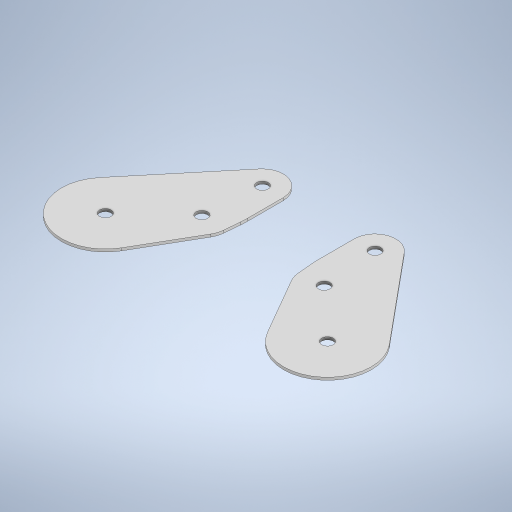
# Autodesk Inventor part: IntakeHolderTopPlate
Saved by Autodesk Inventor 2023 (Build 270158000, 158)
## iProperties
Created: 2022-09-11
Part Number: IntakeHolderTopPlate
Material: Generic
Document SubType Name: Modeling
Designer: deli
Density: 1 g/cm^3
Appearance: Default
Author: deli
Autodesk Inventor part; units mm, degrees
ref_plane "YZ Plane" through (0, 0, 0) normal (1, 0, 0) x (0, 1, 0)
ref_plane "XZ Plane" through (0, 0, 0) normal (0, 1, 0) x (-1, 0, 0)
ref_plane "XY Plane" through (0, 0, 0) normal (0, 0, 1) x (1, 0, 0)
sketch "Sketch1" plane through (0, 0, 0) normal (0, 1, 0) x (-1, 0, 0)
  circle A0 centre (21.4316, 162.4913) radius 7
  circle A1 centre (21.4316, 162.4913) radius 24 construction
  circle A2 centre (15.5486, 229.7344) radius 24 construction
  circle A3 centre (15.5486, 229.7344) radius 7
  circle A4 centre (157.4316, 162.4913) radius 7
  circle A5 centre (163.3146, 229.7344) radius 7
  circle A6 centre (163.3146, 229.7344) radius 24 construction
  circle A7 centre (157.4316, 162.4913) radius 24 construction
  line L0 (157.4316, 162.4913) -> (21.4316, 162.4913) construction
  line L1 (15.5486, 229.7344) -> (21.4316, 162.4913) construction
  line L2 (163.3146, 229.7344) -> (157.4316, 162.4913) construction
  circle A8 centre (89.4316, 131.3298) radius 50.8 construction
  line L3 (44.4382, 232.2619) -> (46.051, 213.8271)
  line L4 (134.4249, 232.2619) -> (132.8121, 213.8271)
  arc A9 (138.1998, 244.2344) -> (134.4249, 232.2619) centre (163.3146, 229.7344) ccw
  arc A10 (2.1886, 146.5317) -> (46.4316, 162.4913) centre (21.4316, 162.4913) ccw
  arc A11 (132.4316, 162.4913) -> (176.6745, 146.5317) centre (157.4316, 162.4913) ccw
  line L5 (46.4316, 162.4913) -> (46.4316, 205.1116)
  line L6 (132.4316, 162.4913) -> (132.4316, 205.1116)
  arc A12 (46.4316, 205.1116) -> (46.051, 213.8271) centre (-53.5684, 205.1116) ccw
  arc A13 (132.8121, 213.8271) -> (132.4316, 205.1116) centre (232.4316, 205.1116) ccw
  circle A14 centre (-44.702, 286.0915) radius 48 construction
  line L7 (-3.1328, 310.0915) -> (36.3332, 241.7344) construction
  circle A15 centre (-44.702, 286.0915) radius 7
  arc A16 (1.1973, 312.5915) -> (-85.4971, 252.2572) centre (-44.702, 286.0915) ccw
  line L8 (1.1973, 312.5915) -> (40.6633, 244.2344)
  arc A17 (44.4382, 232.2619) -> (40.6633, 244.2344) centre (15.5486, 229.7344) ccw
  line L9 (-85.4971, 252.2572) -> (2.1886, 146.5317)
  circle A18 centre (223.5652, 286.0915) radius 7
  arc A19 (264.3603, 252.2572) -> (177.6658, 312.5915) centre (223.5652, 286.0915) ccw
  circle A20 centre (223.5652, 286.0915) radius 48 construction
  line L10 (181.9959, 310.0915) -> (142.53, 241.7344) construction
  line L11 (177.6658, 312.5915) -> (138.1998, 244.2344)
  line L12 (264.3603, 252.2572) -> (176.6745, 146.5317)
  point P0 (0, 0)
  dimension "d2" = 48
  dimension "d5" = 48
  dimension "d26" = 96
  dimension "d32" = 96
  dimension "d36" = 99.766
  dimension "d0" = 14
  dimension "d1" = 48
  dimension "d3" = 14
  dimension "d4" = 67.5
  dimension "d6" = 14
  dimension "d7" = 14
  dimension "d8" = 48
  dimension "d9" = 67.5
  dimension "d10" = 88
  dimension "d11" = 95
  dimension "d12" = 95
  dimension "d13" = 101.6
  dimension "d18" = 5
  dimension "d19" = 5
  dimension "d21" = 86
  dimension "d22" = 100
  dimension "d23" = 100
  dimension "d27" = 82.5
  dimension "d28" = 120
  dimension "d29" = 14
  dimension "d30" = 5
  dimension "d31" = 14
  dimension "d33" = 5
  dimension "d34" = 120
  dimension "d35" = 82.5
  constraints: 26 end point, 18 tangent, 17 centre point, 16 point on circle, 12 coincident, 2 parallel, 2 vertical, 1 equal radius, 1 horizontal, 1 point on line, 16 other
  measures "d0" diameter of A0
  measures "d1" diameter of A1
  measures "d3" diameter of A3
  measures "d4" distance of A0.centre L1.start
  measures "d6" diameter of A5
  measures "d7" diameter of A4
  measures "d8" diameter of A7
  measures "d9" distance of A4.centre A5.centre
  measures "d11" angle of L0 L2
  measures "d12" angle of L0 L1
  measures "d13" diameter of A8
  measures "d21" distance between parallel lines of L6 L5
  measures "d22" radius of A12
  measures "d23" radius of A13
  measures "d27" distance of point (15.549, 229.734) point (-44.702, 286.091)
  measures "d28" angle of L0 L7
  measures "d29" diameter of A15
  measures "d31" diameter of A18
  measures "d34" angle of L0 L10
  measures "d35" distance of A5.centre A18.centre
extrude "Extrusion1" add sketch "Sketch1" along normal blind 3.175
equation "\"d2\" = d1"
equation "\"d5\" = d1"
equation "\"d32\" = d26"
equation "\"d3\" = d0"
equation "\"d6\" = d0"
equation "\"d7\" = d0"
equation "\"d8\" = d1"
equation "\"d9\" = d4"
equation "\"d12\" = d11"
equation "\"d19\" = d18"
equation "\"d23\" = d22"
equation "\"d30\" = d18"
equation "\"d31\" = d29"
equation "\"d33\" = d30"
equation "\"d34\" = d28"
equation "\"d35\" = d27"
equation "\"d17\" = d16"
equation "\"d16\" = 5"
body "Solid1"
